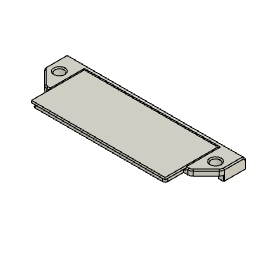
Nameplate Middle Clip (Autodesk Fusion 360 design; units mm, degrees)
Autodesk Fusion 360 part; units mm, degrees
sketch "Sketch1" plane through (0, 0, 0) normal (0, 0, 1) x (1, 0, 0) in component "Nameplate"
  line L0 (25, 10) -> (-25, 10)
  line L1 (-25, 10) -> (-25, -10)
  line L2 (-25, -10) -> (25, -10)
  line L3 (25, -10) -> (25, 10)
  line L4 (25, 10) -> (-25, -10) construction
  line L5 (-25, 10) -> (25, -10) construction
  dimension "d1" = 50
  dimension "d2" = 20
  constraint horizontal L0
  constraint perpendicular L0 L1
  constraint parallel L0 L2
  constraint parallel L1 L3
  constraint coincident L4 origin
  constraint coincident L5 origin
  measures "d1" distance of L1.end L2.end
  measures "d2" distance of L0.start L2.end
extrude "Extrude1" add sketch "Sketch1" against normal blind 1 makes body 1 in component "Nameplate"
fillet "Fillet1" radius 1.5 4 edges at (25, -10, -0.5) (25, 10, -0.5) (-25, 10, -0.5) (-25, -10, -0.5) on bodies 1 in component "Nameplate"
fillet "Fillet2" radius 0.2 1 faces at (7.8333, -3.3333, 0) on bodies 1 in component "Nameplate"
sketch "Sketch1 (2)" plane through (0, 0, -1) normal (0, 0, -1) x (1, 0, 0) in component "Clip"
  arc A0 (-23.5, 10) -> (-25, 8.5) centre (-23.5, 8.5) ccw
  line L0 (-25, 8.5) -> (-25, -8.5) construction
  arc A1 (-25, -8.5) -> (-23.5, -10) centre (-23.5, -8.5) ccw
  line L1 (-23.5, -10) -> (23.5, -10) construction
  arc A2 (23.5, -10) -> (25, -8.5) centre (23.5, -8.5) ccw
  line L2 (25, -8.5) -> (25, 8.5) construction
  arc A3 (25, 8.5) -> (23.5, 10) centre (23.5, 8.5) ccw
  line L3 (23.5, 10) -> (-23.5, 10) construction
  line L4 (-33, -12.25) -> (33, -12.25)
  line L5 (-33, -12.25) -> (-33, -3.25)
  line L6 (-33, -3.25) -> (-27, 2.75)
  line L7 (-27, 2.75) -> (27, 2.75)
  line L8 (27, 2.75) -> (33, -3.25)
  line L9 (33, -3.25) -> (33, -12.25)
  line L10 (-33, -3.75) -> (33, -3.75) construction
  line L11 (0, -10) -> (0, -12.25) construction
  circle A4 centre (-29, -4.75) radius 1.7
  circle A5 centre (29, -4.75) radius 1.7
  line L12 (0, 2.75) -> (0, 10) construction
  line L13 (-29, -4.75) -> (29, -4.75) construction
  line L14 (0, -10) -> (0, -4.75) construction
  line L15 (-24.6, 9.6) -> (24.6, 9.6)
  line L16 (24.6, 9.6) -> (24.6, 2.75)
  line L17 (24.6, 2.75) -> (-24.6, 2.75)
  line L18 (-24.6, 2.75) -> (-24.6, 9.6)
  dimension "d9" = 8.5
  dimension "d10" = 7.5
  dimension "d12" = 3.4
  dimension "d13" = 45
  dimension "d20" = 15
  dimension "d21" = 2.25
  dimension "d22" = 4
  dimension "d23" = 4
  dimension "d24" = 2
  dimension "d35" = 0.4
  dimension "d36" = 0.4
  dimension "d37" = 0.4
  constraint parallel L1 L4
  constraint perpendicular L4 L5
  constraint parallel L4 L7
  constraint perpendicular L7 L9
  constraint coincident L5 L10.start
  constraint coincident L9 L10.end
  constraint perpendicular L9 L10
  constraint midpoint L1 L11.start
  constraint perpendicular L1 L11
  constraint midpoint L4 L11.end
  constraint equal A4 A5
  constraint midpoint L7 L12.start
  constraint perpendicular L7 L12
  constraint midpoint L3 L12.end
  constraint equal L5 L9
  constraint coincident A4.centre L13.start
  constraint coincident A5.centre L13.end
  constraint horizontal L13
  constraint coincident L13 L14.end
  constraint vertical L14
  constraint midpoint L13 L14.end
  constraint horizontal L15
  constraint vertical L16
  constraint horizontal L17
  constraint vertical L18
  constraint coincident L7 L16.end
  measures "d9" distance of L4 L10
  measures "d10" distance of L4 A4.centre
  measures "d12" diameter of A4
  measures "d13" angle of L4 L8
  measures "d20" vertical distance of L4.end L7.end
  measures "d21" distance of L1 L4
  measures "d22" distance of L9 A5.centre
  measures "d23" distance of L2 A5.centre
  measures "d24" distance of L2 L7.end
  measures "d35" distance of L0 L18
  measures "d36" distance of L3 L15
  measures "d37" distance of L2 L16
extrude "Extrude1'" add sketch "Sketch1 (2)" along normal blind 1 separate body makes body 2 in component "Clip"
sketch "Sketch2" plane through (0, 0, -2) normal (0, 0, -1) x (1, 0, 0) in component "Clip"
  circle A0 centre (29, -4.75) radius 1.7
  circle A1 centre (-29, -4.75) radius 1.7
  line L0 (-33, -12.25) -> (33, -12.25)
  line L1 (33, -12.25) -> (33, -3.25)
  line L2 (33, -3.25) -> (27, 2.75)
  line L3 (27, 2.75) -> (24.6, 2.75)
  line L4 (-27, 2.75) -> (-33, -3.25)
  line L5 (-33, -3.25) -> (-33, -12.25)
  line L6 (-33, -3.75) -> (33, -3.75)
  line L7 (30.7, -3.75) -> (30.7, -4.75)
  line L8 (27.3, -3.75) -> (27.3, -4.75)
  line L9 (-30.7, -3.75) -> (-30.7, -4.75)
  line L10 (-27.3, -3.75) -> (-27.3, -4.75)
  line L11 (24.6, 2.75) -> (24.6, 9.6)
  line L12 (24.6, 9.6) -> (-24.6, 9.6)
  line L13 (-24.6, 9.6) -> (-24.6, 2.75)
  line L14 (-24.6, 2.75) -> (-27, 2.75)
  dimension "d16" = 8.5
  constraint coincident L5 L6.start
  constraint coincident L1 L6.end
  constraint perpendicular L1 L6
  constraint coincident L6 L7.start
  constraint perpendicular L6 L7
  constraint coincident L6 L8.start
  constraint perpendicular L6 L8
  constraint coincident L6 L9.start
  constraint perpendicular L6 L9
  constraint coincident L6 L10.start
  constraint perpendicular L6 L10
  constraint coincident A1 L9.end
  constraint coincident A1 L10.end
  constraint coincident A0 L8.end
  constraint coincident A0 L7.end
  constraint tangent A1 L9
  constraint tangent A1 L10
  constraint tangent A0 L8
  constraint tangent A0 L7
  measures "d16" distance of L0.end L6.end
extrude "Extrude2" add sketch "Sketch2" along normal blind 2 contours A0 A1 L0 L1 L5 L6 L7 L8 L9 L10 bodies 2 in component "Clip"
chamfer "Chamfer1" distance 0.4 angle 45 4 edges at (-30.7, 3.75, -3) (-27.3, 3.75, -3) (27.3, 3.75, -3) (30.7, 3.75, -3) on bodies 2 in component "Clip"
sketch "Sketch3" plane through (0, 0, -1) normal (0, 0, 1) x (-1, 0, 0) in component "Clip"
  circle A0 centre (-29, -4.75) radius 1.7
  circle A1 centre (29, -4.75) radius 1.7
  line L0 (-33, -12.25) -> (33, -12.25)
  line L1 (33, -12.25) -> (33, -3.25)
  line L2 (33, -3.25) -> (27, 2.75)
  line L3 (27, 2.75) -> (24.6, 2.75)
  line L4 (-27, 2.75) -> (-33, -3.25)
  line L5 (-33, -3.25) -> (-33, -12.25)
  line L6 (25, 8.5) -> (25, -8.5)
  line L7 (-25, -8.5) -> (-25, 8.5)
  line L8 (23.5, -10) -> (-23.5, -10)
  line L9 (-25.25, 2.75) -> (-25.25, -10.25)
  line L10 (-25.25, -10.25) -> (25.25, -10.25)
  line L11 (25.25, -10.25) -> (25.25, 2.75)
  line L12 (24.6, 2.75) -> (24.6, 9.6)
  line L13 (24.6, 9.6) -> (-24.6, 9.6)
  line L14 (-24.6, 9.6) -> (-24.6, 2.75)
  line L15 (-24.6, 2.75) -> (-27, 2.75)
  dimension "d25" = 0.25
  dimension "d26" = 0.25
  dimension "d27" = 0.25
  constraint coincident L3 L9.start
  constraint perpendicular L3 L9
  constraint perpendicular L9 L10
  constraint perpendicular L10 L11
  constraint coincident L3 L11.end
  measures "d25" distance of L6 L11
  measures "d26" distance of L7 L9.start
  measures "d27" distance of L8 L10
extrude "Extrude3" add sketch "Sketch3" along normal blind 1 contours L0 L1 L2 L3 L4 L5 L9 L10 L11 L15 bodies 2 in component "Clip"
fillet "Fillet1'" radius 2 4 edges at (-27, -2.75, -1) (-33, 3.25, -1) (33, 3.25, -1) (27, -2.75, -1) on bodies 2 in component "Clip"
chamfer "Chamfer2" distance 1 angle 45 1 edges at (0, 12.25, 0) on bodies 2 in component "Clip"
fillet "Fillet2'" radius 1 2 edges at (-24.6, -9.6, -1.5) (24.6, -9.6, -1.5) on bodies 2 in component "Clip"
chamfer "Chamfer4" distance 0.4 angle 45 16 edges at (26.9369, -2.5978, 0) (30, 0.25, 0) (32.8478, 3.3131, 0) (33, 7.6642, 0) (25.7108, -2.75, 0) (-30, 0.25, 0) (-32.8478, 3.3131, 0) (-33, 7.6642, 0) (-25.7108, -2.75, 0) (-26.9369, -2.5978, 0) (-33, 11.75, -0.5) (33, 11.75, -0.5) (33, 12.25, -2.5) (-33, 12.25, -2.5) (30.585, 4.1353, 0) (-27.415, 4.1353, 0) on bodies 2 in component "Clip"
sketch "Sketch4" plane through (0, 0, 0) normal (0, 0, 1) x (-1, 0, 0) in component "Clip"
  circle A0 centre (-29, -4.75) radius 2.1
  line L0 (26.1716, 2.35) -> (25.25, 2.35)
  line L1 (25.25, 2.35) -> (25.25, -10.25)
  line L2 (25.25, -10.25) -> (-25.25, -10.25)
  line L3 (-25.25, -10.25) -> (-25.25, 2.35)
  line L4 (-25.25, 2.35) -> (-26.1716, 2.35)
  arc A1 (-26.1716, 2.35) -> (-27.3029, 1.8814) centre (-26.1716, 0.75) ccw
  line L5 (-27.3029, 1.8814) -> (-32.1314, -2.9471)
  arc A2 (-32.1314, -2.9471) -> (-32.6, -4.0784) centre (-31, -4.0784) ccw
  line L6 (-32.6, -4.0784) -> (-32.6, -11.25)
  line L7 (-32.6, -11.25) -> (32.6, -11.25)
  line L8 (32.6, -11.25) -> (32.6, -4.0784)
  arc A3 (32.6, -4.0784) -> (32.1314, -2.9471) centre (31, -4.0784) ccw
  line L9 (32.1314, -2.9471) -> (27.3029, 1.8814)
  arc A4 (27.3029, 1.8814) -> (26.1716, 2.35) centre (26.1716, 0.75) ccw
  circle A5 centre (29, -4.75) radius 2.1
  line L10 (-24.8, -9.8) -> (24.8, -9.8)
  line L11 (24.8, -9.8) -> (24.8, 9.8)
  line L12 (24.8, 9.8) -> (-24.8, 9.8)
  line L13 (-24.8, 9.8) -> (-24.8, -9.8)
  line L14 (-24.8, -9.8) -> (24.8, 9.8) construction
  line L15 (24.8, -9.8) -> (-24.8, 9.8) construction
  dimension "d40" = 49.6
  dimension "d41" = 19.6
  constraint horizontal L10
  constraint perpendicular L10 L11
  constraint parallel L10 L12
  constraint parallel L11 L13
  constraint coincident L14 origin
  constraint coincident L15 origin
  measures "d40" distance of L11.end L12.end
  measures "d41" distance of L10.start L12.end
extrude "Extrude4" add sketch "Sketch4" against normal up to surface (0.8 mm away) separate body contours L10 L11 L12 L13 makes body 3 in component "Clip"
component "Nameplate" placed x (1, 0, 0) y (0, 1, 0) z (0, 0, 1) at (0, 0, 0)
component "Clip" placed x (1, 0, 0) y (0, 1, 0) z (0, 0, 1) at (0, 0, 0)
